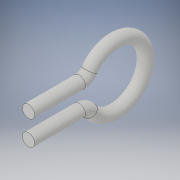
# Autodesk Inventor part: 示範一
Saved by Autodesk Inventor 2017 (Build 210142000, 142)
## iProperties
Part Number: 示範一
Material: 一般
Document SubType Name: Modeling
Designer: user
Density: 1 g/cm^3
Appearance: 預設
Author: user
Autodesk Inventor part; units mm, degrees
ref_plane "YZ Plane" through (0, 0, 0) normal (1, 0, 0) x (0, 1, 0)
ref_plane "XZ Plane" through (0, 0, 0) normal (0, 1, 0) x (-1, 0, 0)
sketch "草圖1" plane through (0, 0, 0) normal (1, 0, 0) x (0, 1, 0)
  arc A0 (-14.2857, 20.5163) -> (14.2857, 20.5163) centre (0, 0) ccw
  line L0 (-10, 28.7228) -> (-10, 70)
  line L1 (0, 0) -> (0, 31.1986)
  line L2 (10, 28.7228) -> (10, 70)
  arc A1 (10, 28.7228) -> (14.2857, 20.5163) centre (20, 28.7228) ccw
  arc A2 (-14.2857, 20.5163) -> (-10, 28.7228) centre (-20, 28.7228) ccw
  point P0 (10, 22.9129)
  point P1 (-10, 22.9129)
  dimension "d0" = 50
  dimension "d1" = 20
  dimension "d2" = 10
  dimension "d4" = 70
  constraints: 8 point on circle, 6 end point, 4 tangent, 3 centre point, 2 point on line, 2 symmetric about line, 2 vertical, 1 coincident, 1 equal radius
  measures "d0" diameter of A0
  measures "d1" distance between parallel lines of L0 L2
  measures "d2" radius of A1
  measures "d4" vertical distance of L2.end point (0, 0)
ref_plane "工作平面1" through (0, 10, 70) normal (0, 0, 1) x (1, 0, 0)
sketch "草圖3" plane through (0, 10, 70) normal (0, 0, 1) x (1, 0, 0)
  circle A0 centre (0, 0) radius 5
  point P0 (0, -10)
  dimension "d3" = 10
  constraints: 1 centre point
  measures "d3" diameter of A0
sweep "掃掠1" add profiles "草圖3" path "草圖1" path curves L2 A1 A0 A2 L0
